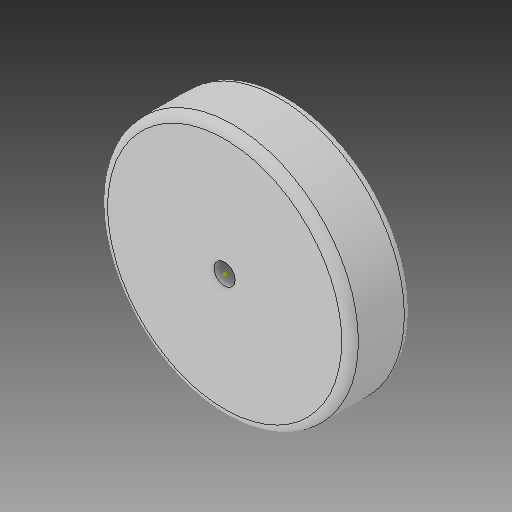
# Autodesk Inventor part: 6 inch wheel
Saved by Autodesk Inventor 2019 (Build 230136000, 136)
## iProperties
Created: 2017-12-07
Part Number: 6 inch wheel
Material: Generic
Document SubType Name: Modeling
Designer: Administrator
Density: 1 g/cm^3
Appearance: Default
Author: Administrator
Autodesk Inventor part; units mm, degrees
ref_plane "YZ Plane" through (0, 0, 0) normal (1, 0, 0) x (0, 1, 0)
ref_plane "XZ Plane" through (0, 0, 0) normal (0, 1, 0) x (-1, 0, 0)
ref_plane "XY Plane" through (0, 0, 0) normal (0, 0, 1) x (1, 0, 0)
sketch "Sketch1" plane through (0, 0, 0) normal (0, 0, 1) x (1, 0, 0)
  circle A0 centre (0, 0) radius 76.2
  dimension "d0" = 152.4
  constraints: 1 centre point, 1 coincident
  measures "d0" diameter of A0
extrude "Extrusion1" add sketch "Sketch1" along normal blind 38.1
sketch "Sketch2" plane through (0, 0, 38.1) normal (0, 0, 1) x (1, 0, 0)
  circle A0 centre (0, 0) radius 6.35
  dimension "d3" = 12.7
  constraints: 1 centre point, 1 coincident
  measures "d3" diameter of A0
extrude "Extrusion2" cut sketch "Sketch2" against normal blind 38.1
sketch "Sketch3" plane through (0, 0, 38.1) normal (0, 0, 1) x (1, 0, 0)
  point P0 (0, 0)
fillet "Fillet1" radius 5.08 2 edges at (-76.2, 0, 38.1) (-76.2, 0, 0)
body "Solid1"
